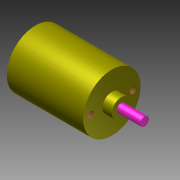
# Autodesk Inventor part: Motor Sensor
Saved by Autodesk Inventor 2012 SP1 (Build 160190100, 190)
## iProperties
Created: 2014-02-18
Part Number: Motor Sensor
Material: Default
Document SubType Name: Modeling
Designer: Pinkponk
Density: 1 g/cm^3
Author: Pinkponk
Autodesk Inventor part; units mm, degrees
ref_plane "YZ Plane" through (0, 0, 0) normal (1, 0, 0) x (0, 1, 0)
ref_plane "XZ Plane" through (0, 0, 0) normal (0, 1, 0) x (-1, 0, 0)
ref_plane "XY Plane" through (0, 0, 0) normal (0, 0, 1) x (1, 0, 0)
sketch "Sketch1" plane through (0, 0, 0) normal (0, 0, 1) x (1, 0, 0)
  line L0 (0, 0) -> (0, 13.5)
  line L1 (0, 13.5) -> (36, 13.5)
  line L2 (36, 13.5) -> (36, 4.4)
  line L3 (36, 4.4) -> (40.4, 4.4)
  line L4 (40.4, 4.4) -> (40.4, 0)
  line L5 (40.4, 0) -> (0, 0)
  line L6 (0, 0) -> (68.0723, 0)
  dimension "d0" = 27
  dimension "d1" = 36
  dimension "d2" = 8.8
  dimension "d3" = 4.4
  constraints: 14 end point, 4 parallel, 1 collinear, 1 perpendicular, 1 vertical
  measures "d0" diameter of L1 L6
  measures "d1" distance of L0.end L1.end
  measures "d2" diameter of L3 L6
  measures "d3" distance of L2.end L3.end
revolve "Revolution1" add sketch "Sketch1" angle 360 about axis through (0, 0, 0) along (1, 0, 0)
sketch "Sketch2" plane through (40.4, 0, 0) normal (1, 0, 0) x (0, 0, -1)
  circle A0 centre (0, 0) radius 4.4 projected
  circle A1 centre (0, 0) radius 2.05
  dimension "d5" = 4.1
  constraints: 1 centre point, 1 coincident
  measures "d5" diameter of A1
extrude "Extrusion1" add sketch "Sketch2" along normal blind 11 contours A1
sketch "Sketch3" plane through (36, 0, 0) normal (1, 0, 0) x (0, 0, -1)
  circle A0 centre (0, 0) radius 4.4 projected
  circle A1 centre (0, 10) radius 1.5
  circle A2 centre (0, -10) radius 1.5
  dimension "d8" = 3
  dimension "d9" = 3
  dimension "d10" = 20
  dimension "d11" = 10
  constraints: 2 centre point, 2 vertical alignment
  measures "d8" diameter of A1
  measures "d9" diameter of A2
  measures "d10" distance of A2.centre A1.centre
  measures "d11" distance of A0.centre A1.centre
extrude "Extrusion2" cut sketch "Sketch3" against normal blind 5 contours A1 | A2
body "Solid1"
